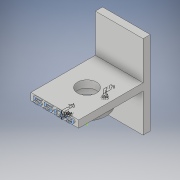
# Autodesk Inventor part: RSL mount
Saved by Autodesk Inventor 2019 (Build 230136000, 136)
## iProperties
Created: 2019-02-11
Part Number: RSL mount
Material: Generic
Document SubType Name: Modeling
Designer: josh
Density: 1 g/cm^3
Appearance: Default
Author: josh
Autodesk Inventor part; units mm, degrees
ref_plane "XZ Plane" through (0, 0, 0) normal (0, 1, 0) x (-1, 0, 0)
ref_plane "XY Plane" through (0, 0, 0) normal (0, 0, 1) x (1, 0, 0)
sketch "Sketch1" plane through (0, 0, 0) normal (0, 0, 1) x (1, 0, 0)
  line L0 (0, 0) -> (50.8, 0)
  line L1 (50.8, 0) -> (50.8, 88.9)
  line L2 (50.8, 88.9) -> (0, 88.9)
  line L3 (0, 88.9) -> (0, 0)
  line L4 (0, 88.9) -> (0, 48.26)
  line L5 (0, 0) -> (0, 40.64)
  line L6 (0, 40.64) -> (50.8, 40.64)
  line L7 (50.8, 48.26) -> (0, 48.26)
  dimension "d0" = 50.8
  dimension "d1" = 88.9
  dimension "d2" = 40.64
  dimension "d3" = 40.64
  constraints: 16 end point, 4 point on line, 3 perpendicular, 2 parallel, 1 horizontal
  measures "d0" distance of L2.end L1.end
  measures "d1" distance of L1.end L0.end
  measures "d2" distance of L2.end L4.end
  measures "d3" distance of L0.start L5.end
extrude "Extrusion1" add sketch "Sketch1" along normal blind 7.62
extrude "Extrusion2" add sketch "Sketch1" along normal blind 76.2 contours L3 L7 L1 L6
sketch "Sketch3" plane through (0, 48.26, 7.62) normal (0, 1, 0) x (1, 0, 0)
  line L0 (0, 0) -> (0, -68.58) projected
  line L1 (0, -34.29) -> (50.8, -34.29)
  line L2 (50.8, 0) -> (50.8, -68.58) projected
  circle A0 centre (25.4, -34.29) radius 10.16
  point P0 (0, 7.62)
  dimension "d8" = 20.32
  constraints: 3 midpoint, 2 end point, 1 centre point
  measures "d8" diameter of A0
extrude "Extrusion3" cut sketch "Sketch3" against normal blind 50.8
sketch "Sketch4" plane through (0, 0, 76.2) normal (0, 0, 1) x (1, 0, 0)
  line L0 (2.1147, 47.7276) -> (47.8791, 47.7276) construction
  line L1 (47.8791, 47.7276) -> (47.8791, 41.3797) construction
  line L2 (47.8791, 41.3797) -> (2.1147, 41.3797) construction
  line L3 (2.1147, 41.3797) -> (2.1147, 47.7276) construction
  spline S0 degree 2 poles (12.464, 43.4446) (12.464, 43.005) (11.7576, 42.2541) (11.1253, 41.9774) knots 0 0 0 1 2 2 2
  spline S1 degree 2 poles (11.1253, 41.9774) (10.4781, 41.7008) (8.5664, 41.3797) (7.3758, 41.3797) knots 0 0 0 1 2 2 2
  spline S2 degree 2 poles (7.3758, 41.3797) (6.2791, 41.3797) (4.1598, 41.5724) (3.3843, 41.7255) knots 0 0 0 1 2 2 2
  line L4 (3.3843, 41.7255) -> (3.3843, 42.59)
  line L5 (3.3843, 42.59) -> (3.5275, 42.59)
  spline S3 degree 2 poles (3.5275, 42.59) (3.7646, 42.5208) (4.644, 42.343) (5.1775, 42.264) knots 0 0 0 1 2 2 2
  spline S4 degree 2 poles (5.1775, 42.264) (5.7802, 42.18) (6.783, 42.0861) (7.4054, 42.0861) knots 0 0 0 1 2 2 2
  spline S5 degree 2 poles (7.4054, 42.0861) (8.018, 42.0861) (9.1888, 42.264) (9.6087, 42.4566) knots 0 0 0 1 2 2 2
  spline S6 degree 2 poles (9.6087, 42.4566) (9.9841, 42.6394) (10.3843, 43.1235) (10.3843, 43.4496) knots 0 0 0 1 2 2 2
  spline S7 degree 2 poles (10.3843, 43.4496) (10.3843, 43.7756) (9.9446, 44.1906) (9.5247, 44.3289) knots 0 0 0 1 2 2 2
  spline S8 degree 2 poles (9.5247, 44.3289) (9.0851, 44.482) (7.8056, 44.6105) (7.0152, 44.6105) knots 0 0 0 1 2 2 2
  spline S9 degree 2 poles (7.0152, 44.6105) (6.1853, 44.6105) (4.5106, 44.5067) (4.0067, 44.4623) knots 0 0 0 1 2 2 2
  line L6 (4.0067, 44.4623) -> (4.0067, 47.6041)
  line L7 (4.0067, 47.6041) -> (12.3702, 47.6041)
  line L8 (12.3702, 47.6041) -> (12.3702, 46.8878)
  line L9 (12.3702, 46.8878) -> (5.9827, 46.8878)
  line L10 (5.9827, 46.8878) -> (5.9827, 45.2626)
  spline S10 degree 2 poles (5.9827, 45.2626) (6.3532, 45.2823) (7.0695, 45.2971) (7.3659, 45.2971) knots 0 0 0 1 2 2 2
  spline S11 degree 2 poles (7.3659, 45.2971) (8.5318, 45.2971) (10.1521, 45.144) (10.898, 44.9168) knots 0 0 0 1 2 2 2
  spline S12 degree 2 poles (10.898, 44.9168) (11.6539, 44.6895) (12.464, 43.9979) (12.464, 43.4446) knots 0 0 0 1 2 2 2
  spline S13 degree 2 poles (23.9052, 43.4446) (23.9052, 43.005) (23.1987, 42.2541) (22.5664, 41.9774) knots 0 0 0 1 2 2 2
  spline S14 degree 2 poles (22.5664, 41.9774) (21.9193, 41.7008) (20.0075, 41.3797) (18.8169, 41.3797) knots 0 0 0 1 2 2 2
  spline S15 degree 2 poles (18.8169, 41.3797) (17.7202, 41.3797) (15.601, 41.5724) (14.8254, 41.7255) knots 0 0 0 1 2 2 2
  line L11 (14.8254, 41.7255) -> (14.8254, 42.59)
  line L12 (14.8254, 42.59) -> (14.9686, 42.59)
  spline S16 degree 2 poles (14.9686, 42.59) (15.2058, 42.5208) (16.0851, 42.343) (16.6186, 42.264) knots 0 0 0 1 2 2 2
  spline S17 degree 2 poles (16.6186, 42.264) (17.2213, 42.18) (18.2241, 42.0861) (18.8466, 42.0861) knots 0 0 0 1 2 2 2
  spline S18 degree 2 poles (18.8466, 42.0861) (19.4591, 42.0861) (20.6299, 42.264) (21.0498, 42.4566) knots 0 0 0 1 2 2 2
  spline S19 degree 2 poles (21.0498, 42.4566) (21.4253, 42.6394) (21.8254, 43.1235) (21.8254, 43.4496) knots 0 0 0 1 2 2 2
  spline S20 degree 2 poles (21.8254, 43.4496) (21.8254, 43.7756) (21.3857, 44.1906) (20.9658, 44.3289) knots 0 0 0 1 2 2 2
  spline S21 degree 2 poles (20.9658, 44.3289) (20.5262, 44.482) (19.2467, 44.6105) (18.4563, 44.6105) knots 0 0 0 1 2 2 2
  spline S22 degree 2 poles (18.4563, 44.6105) (17.6264, 44.6105) (15.9517, 44.5067) (15.4478, 44.4623) knots 0 0 0 1 2 2 2
  line L13 (15.4478, 44.4623) -> (15.4478, 47.6041)
  line L14 (15.4478, 47.6041) -> (23.8113, 47.6041)
  line L15 (23.8113, 47.6041) -> (23.8113, 46.8878)
  line L16 (23.8113, 46.8878) -> (17.4238, 46.8878)
  line L17 (17.4238, 46.8878) -> (17.4238, 45.2626)
  spline S23 degree 2 poles (17.4238, 45.2626) (17.7943, 45.2823) (18.5106, 45.2971) (18.807, 45.2971) knots 0 0 0 1 2 2 2
  spline S24 degree 2 poles (18.807, 45.2971) (19.9729, 45.2971) (21.5932, 45.144) (22.3392, 44.9168) knots 0 0 0 1 2 2 2
  spline S25 degree 2 poles (22.3392, 44.9168) (23.095, 44.6895) (23.9052, 43.9979) (23.9052, 43.4446) knots 0 0 0 1 2 2 2
  spline S26 degree 2 poles (35.5883, 44.5561) (35.5883, 42.9161) (33.2023, 41.3797) (30.7175, 41.3797) knots 0 0 0 1 2 2 2
  spline S27 degree 2 poles (30.7175, 41.3797) (28.198, 41.3797) (25.8466, 42.9457) (25.8466, 44.5512) knots 0 0 0 1 2 2 2
  spline S28 degree 2 poles (25.8466, 44.5512) (25.8466, 46.2012) (28.2326, 47.7276) (30.7175, 47.7276) knots 0 0 0 1 2 2 2
  spline S29 degree 2 poles (30.7175, 47.7276) (33.2369, 47.7276) (35.5883, 46.1468) (35.5883, 44.5561) knots 0 0 0 1 2 2 2
  spline S30 degree 2 poles (32.9652, 42.6987) (33.2616, 43) (33.5086, 43.9288) (33.5086, 44.5561) knots 0 0 0 1 2 2 2
  spline S31 degree 2 poles (33.5086, 44.5561) (33.5086, 45.1835) (33.2616, 46.1073) (32.9553, 46.4185) knots 0 0 0 1 2 2 2
  spline S32 degree 2 poles (32.9553, 46.4185) (32.649, 46.7298) (31.577, 47.0509) (30.7175, 47.0509) knots 0 0 0 1 2 2 2
  spline S33 degree 2 poles (30.7175, 47.0509) (29.8678, 47.0509) (28.776, 46.7298) (28.4599, 46.4087) knots 0 0 0 1 2 2 2
  spline S34 degree 2 poles (28.4599, 46.4087) (28.1536, 46.0974) (27.9263, 45.1489) (27.9263, 44.5512) knots 0 0 0 1 2 2 2
  spline S35 degree 2 poles (27.9263, 44.5512) (27.9263, 43.909) (28.119, 43.0494) (28.45, 42.7135) knots 0 0 0 1 2 2 2
  spline S36 degree 2 poles (28.45, 42.7135) (28.7464, 42.3973) (29.8381, 42.0565) (30.7175, 42.0565) knots 0 0 0 1 2 2 2
  spline S37 degree 2 poles (30.7175, 42.0565) (31.5671, 42.0565) (32.6589, 42.3776) (32.9652, 42.6987) knots 0 0 0 1 2 2 2
  spline S38 degree 2 poles (37.1247, 45.6232) (37.1247, 46.0925) (37.8904, 46.873) (38.5573, 47.1546) knots 0 0 0 1 2 2 2
  spline S39 degree 2 poles (38.5573, 47.1546) (39.1896, 47.4263) (41.0224, 47.7276) (41.9659, 47.7276) knots 0 0 0 1 2 2 2
  spline S40 degree 2 poles (41.9659, 47.7276) (43.0181, 47.7276) (44.7274, 47.4461) (45.3498, 47.1793) knots 0 0 0 1 2 2 2
  spline S41 degree 2 poles (45.3498, 47.1793) (46.1402, 46.8434) (47.0097, 45.7566) (47.0097, 44.9217) knots 0 0 0 1 2 2 2
  spline S42 degree 2 poles (47.0097, 44.9217) (47.0097, 44.1659) (46.16, 42.8123) (45.3301, 42.3628) knots 0 0 0 1 2 2 2
  spline S43 degree 2 poles (45.3301, 42.3628) (44.4507, 41.8885) (41.9857, 41.3896) (40.1727, 41.3896) knots 0 0 0 1 2 2 2
  spline S44 degree 2 poles (40.1727, 41.3896) (39.7627, 41.3896) (38.8438, 41.4242) (38.4437, 41.4736) knots 0 0 0 1 2 2 2
  line L18 (38.4437, 41.4736) -> (38.4437, 42.259)
  line L19 (38.4437, 42.259) -> (38.5474, 42.259)
  spline S45 degree 2 poles (38.5474, 42.259) (38.8043, 42.1997) (39.8862, 42.096) (40.4493, 42.096) knots 0 0 0 1 2 2 2
  spline S46 degree 2 poles (40.4493, 42.096) (42.455, 42.096) (44.7521, 43.1532) (44.9052, 44.1313) knots 0 0 0 1 2 2 2
  spline S47 degree 2 poles (44.9052, 44.1313) (44.0852, 43.909) (42.5982, 43.7065) (41.7288, 43.7065) knots 0 0 0 1 2 2 2
  spline S48 degree 2 poles (41.7288, 43.7065) (40.8791, 43.7065) (39.491, 43.8547) (38.7845, 44.0671) knots 0 0 0 1 2 2 2
  spline S49 degree 2 poles (38.7845, 44.0671) (37.9645, 44.319) (37.1247, 45.0847) (37.1247, 45.6232) knots 0 0 0 1 2 2 2
  spline S50 degree 2 poles (44.9546, 45.1045) (44.9546, 45.722) (44.3816, 46.5025) (43.8826, 46.7149) knots 0 0 0 1 2 2 2
  spline S51 degree 2 poles (43.8826, 46.7149) (43.4282, 46.9125) (42.5093, 47.0607) (41.956, 47.0607) knots 0 0 0 1 2 2 2
  spline S52 degree 2 poles (41.956, 47.0607) (40.6963, 47.0607) (39.2044, 46.3395) (39.2044, 45.6578) knots 0 0 0 1 2 2 2
  spline S53 degree 2 poles (39.2044, 45.6578) (39.2044, 45.2724) (39.6935, 44.7735) (40.2468, 44.5957) knots 0 0 0 1 2 2 2
  spline S54 degree 2 poles (40.2468, 44.5957) (40.637, 44.4672) (41.6201, 44.3832) (42.1833, 44.3832) knots 0 0 0 1 2 2 2
  spline S55 degree 2 poles (42.1833, 44.3832) (42.8354, 44.3832) (44.3519, 44.566) (44.9151, 44.7192) knots 0 0 0 1 2 2 2
  spline S56 degree 2 poles (44.9151, 44.7192) (44.925, 44.7784) (44.9546, 44.981) (44.9546, 45.1045) knots 0 0 0 1 2 2 2
  point P0 (0, 0)
  constraints: 2 other
emboss "Emboss1" sketch "Sketch4" operation add depth 1.27 direction (0, 0, -1)
ref_plane "Work Plane1" through (25.4, 0, 0) normal (1, 0, 0) x (0, 1, 0)
sketch "Sketch5" plane through (25.4, 0, 0) normal (1, 0, 0) x (0, 1, 0)
  line L0 (40.64, 56.014) -> (32.131, 56.014)
  line L1 (40.64, 27.806) -> (32.131, 27.806)
  line L2 (40.64, 56.014) -> (40.64, 62.364)
  line L3 (32.131, 62.364) -> (32.131, 56.014)
  line L4 (32.131, 27.806) -> (32.131, 21.456)
  line L5 (32.131, 62.364) -> (36.3855, 62.364)
  line L6 (36.3855, 62.364) -> (36.3855, 61.094)
  line L7 (36.3855, 61.094) -> (33.8455, 61.094)
  line L8 (33.8455, 61.094) -> (33.8455, 59.189)
  line L9 (33.8455, 59.189) -> (38.1635, 59.189)
  line L10 (38.1635, 59.189) -> (38.1635, 62.364)
  line L11 (38.1635, 21.456) -> (38.1635, 24.631)
  line L12 (38.1635, 24.631) -> (33.8455, 24.631)
  line L13 (33.8455, 24.631) -> (33.8455, 22.726)
  line L14 (33.8455, 22.726) -> (36.3855, 22.726)
  line L15 (36.3855, 22.726) -> (36.3855, 21.456)
  line L16 (40.64, 41.91) -> (13.3619, 41.91)
  line L17 (40.64, 21.456) -> (38.1635, 21.456)
  line L18 (36.3855, 21.456) -> (32.131, 21.456)
  line L19 (40.64, 62.364) -> (38.1635, 62.364)
  line L20 (36.3855, 62.364) -> (32.131, 62.364)
  line L21 (40.64, 21.456) -> (40.64, 27.806)
  point P0 (0, 0)
  dimension "d15" = 8.509
  dimension "d18" = 6.35
  dimension "d19" = 1.27
  dimension "d20" = 2.54
  dimension "d21" = 4.318
  dimension "d22" = 3.175
  dimension "d23" = 4.318
  dimension "d25" = 1.27
  constraints: 44 end point, 8 perpendicular, 3 vertical, 2 horizontal, 1 collinear, 1 parallel
  measures "d15" distance of L0.start L0.end
  measures "d18" distance of L0.start L2.end
  measures "d19" distance of L5.end L6.end
  measures "d20" distance of L6.end L7.end
  measures "d21" distance of L8.end L9.end
  measures "d22" distance of L11.start L11.end
  measures "d23" distance of L11.end L12.end
  measures "d25" distance of L14.end L15.end
revolve "Revolution1" add sketch "Sketch5" angle 15 about axis through (25.4, 40.64, 41.91) along (0, -1, 0)
ref_plane "Work Plane2" through (20.1061, 38.1635, 61.667) normal (-0.9659258, 0, -0.258819) x (0, -1, 0)
sketch "Sketch6" plane through (20.1061, 38.1635, 61.667) normal (-0.9659258, 0, -0.258819) x (0, -1, 0)
  line L0 (-2.4765, -6.35) -> (-2.4765, 0) projected
  line L1 (-2.4765, -6.35) -> (6.0325, -6.35) projected
  line L2 (6.0325, -6.35) -> (6.0325, 0) projected
  line L3 (6.0325, 0) -> (1.778, 0) projected
  line L4 (1.778, 0) -> (1.778, -1.27) projected
  line L5 (1.778, -1.27) -> (4.318, -1.27) projected
  line L6 (4.318, -1.27) -> (4.318, -3.175) projected
  line L7 (4.318, -3.175) -> (0, -3.175) projected
  line L8 (0, -3.175) -> (0, 0) projected
  line L9 (0, 0) -> (-2.4765, 0) projected
  line L10 (1.778, 0) -> (1.778, -1.27) projected
  line L11 (1.778, -1.27) -> (1.778, -3.175)
  line L12 (1.778, 0) -> (1.778, -1.27)
  line L13 (-2.4765, -6.35) -> (6.0325, -6.35)
  line L14 (6.0325, -6.35) -> (6.0325, 0)
  line L15 (-2.4765, 0) -> (-2.4765, -6.35)
  line L16 (6.0325, 0) -> (1.778, 0)
  line L17 (0, 0) -> (-2.4765, 0)
  line L18 (0, -3.175) -> (0, 0) projected
  line L19 (1.778, -3.175) -> (0, -3.175)
  line L20 (0, -3.175) -> (0, 0)
  line L21 (-2.4765, -34.558) -> (6.0325, -34.558) projected
  line L22 (6.0325, -34.558) -> (6.0325, -40.908) projected
  line L23 (6.0325, -40.908) -> (1.778, -40.908) projected
  line L24 (1.778, -40.908) -> (1.778, -39.638) projected
  line L25 (1.778, -39.638) -> (4.318, -39.638) projected
  line L26 (4.318, -39.638) -> (4.318, -37.733) projected
  line L27 (4.318, -37.733) -> (0, -37.733) projected
  line L28 (0, -37.733) -> (0, -40.908) projected
  line L29 (0, -40.908) -> (-2.4765, -40.908) projected
  line L30 (-2.4765, -34.558) -> (-2.4765, -40.908) projected
  line L31 (1.778, -40.908) -> (1.778, -37.733)
  line L32 (4.318, -37.733) -> (0, -37.733) projected
  line L33 (1.778, -37.733) -> (0, -37.733)
  line L34 (0, -37.733) -> (0, -40.908)
  line L35 (-2.4765, -34.558) -> (6.0325, -34.558)
  line L36 (6.0325, -34.558) -> (6.0325, -40.908)
  line L37 (-2.4765, -40.908) -> (-2.4765, -34.558)
  line L38 (6.0325, -40.908) -> (1.778, -40.908)
  line L39 (0, -40.908) -> (-2.4765, -40.908)
  line L40 (-2.4765, 0) -> (-2.4765, -40.908)
  line L41 (-2.4765, -47.0016) -> (-2.4765, 19.2416) projected
  line L42 (-2.4765, -20.454) -> (9.1387, -20.454)
  point P0 (38.1635, -54.3619)
  constraints: 39 end point, 6 parallel, 6 perpendicular, 4 horizontal, 2 collinear, 2 point on line, 1 midpoint, 1 vertical
revolve "Revolution2" add sketch "Sketch6" angle 20 about axis through (25.4, 40.64, 41.91) along (0, -1, 0)
ref_plane "Work Plane3" through (25.4, 36.3855, 62.364) normal (-1, 0, 0) x (0, -1, 0)
sketch "Sketch7" plane through (25.4, 36.3855, 62.364) normal (-1, 0, 0) x (0, -1, 0)
  line L0 (-4.2545, 0) -> (-4.2545, -6.35) projected
  line L1 (-4.2545, 0) -> (-1.778, 0) projected
  line L2 (0, 0) -> (4.2545, 0) projected
  line L3 (4.2545, 0) -> (4.2545, -6.35) projected
  line L4 (4.2545, -6.35) -> (-4.2545, -6.35) projected
  line L5 (-4.2545, -34.558) -> (4.2545, -34.558) projected
  line L6 (-4.2545, -40.908) -> (-4.2545, -34.558) projected
  line L7 (-1.778, -40.908) -> (-4.2545, -40.908) projected
  line L8 (4.2545, -40.908) -> (0, -40.908) projected
  line L9 (4.2545, -34.558) -> (4.2545, -40.908) projected
  line L10 (-4.2545, 0) -> (4.2545, 0)
  line L11 (4.2545, 0) -> (4.2545, -6.35)
  line L12 (4.2545, -6.35) -> (-4.2545, -6.35)
  line L13 (-4.2545, -6.35) -> (-4.2545, 0)
  line L14 (-4.2545, -40.908) -> (4.2545, -40.908)
  line L15 (4.2545, -40.908) -> (4.2545, -34.558)
  line L16 (4.2545, -34.558) -> (-4.2545, -34.558)
  line L17 (-4.2545, -34.558) -> (-4.2545, -40.908)
  line L18 (-4.2545, -40.908) -> (-4.2545, 0)
  line L19 (-4.2545, -20.454) -> (4.2545, -20.454)
  point P0 (36.3855, -62.364)
  point P1 (-1.778, -3.175)
  constraints: 20 end point, 4 parallel, 3 horizontal, 2 perpendicular, 1 midpoint, 1 vertical
revolve "Revolution3" add sketch "Sketch7" angle 130 about axis through (25.4, 40.64, 41.91) along (0, 1, 0)
ref_plane "Work Plane4" through (13.6681, 36.3855, 58.6649) normal (-0.819152, 0, -0.5735764) x (0, -1, 0)
sketch "Sketch8" plane through (13.6681, 36.3855, 58.6649) normal (-0.819152, 0, -0.5735764) x (0, -1, 0)
  line L0 (0, -3.175) -> (-1.778, -3.175) projected
  line L1 (-1.778, -3.175) -> (-1.778, 0) projected
  line L2 (-1.778, 0) -> (-4.2545, 0) projected
  line L3 (-4.2545, -6.35) -> (-4.2545, 0) projected
  line L4 (-4.2545, -6.35) -> (4.2545, -6.35) projected
  line L5 (4.2545, -6.35) -> (4.2545, 0) projected
  line L6 (4.2545, 0) -> (0, 0) projected
  line L7 (0, 0) -> (0, -3.175) projected
  line L8 (0, -40.908) -> (0, -37.733) projected
  line L9 (0, -37.733) -> (-1.778, -37.733) projected
  line L10 (-1.778, -37.733) -> (-1.778, -40.908) projected
  line L11 (-1.778, -40.908) -> (-4.2545, -40.908) projected
  line L12 (-4.2545, -34.558) -> (-4.2545, -40.908) projected
  line L13 (-4.2545, -34.558) -> (4.2545, -34.558) projected
  line L14 (4.2545, -34.558) -> (4.2545, -40.908) projected
  line L15 (4.2545, -40.908) -> (0, -40.908) projected
  line L16 (-1.778, -37.733) -> (-1.778, -34.6081) projected
  line L17 (-1.778, -37.733) -> (4.2545, -37.733)
  line L18 (4.2545, -34.558) -> (-4.2545, -34.558)
  line L19 (4.2545, -40.908) -> (0, -40.908) projected
  line L20 (-4.2545, -34.558) -> (-4.2545, -40.908) projected
  line L21 (-4.2545, -40.908) -> (-1.778, -40.908)
  line L22 (-1.778, -37.733) -> (-1.778, -40.908)
  line L23 (-4.2545, -6.35) -> (4.2545, -6.35) projected
  line L24 (4.2545, -6.35) -> (-4.2545, -6.35)
  line L25 (-4.2545, -6.35) -> (-4.2545, 0)
  line L26 (-1.778, 0) -> (-1.778, -3.175)
  line L27 (0, -3.175) -> (-1.778, -3.175) projected
  line L28 (-1.778, -3.175) -> (4.2545, -3.175)
  line L29 (4.2545, -6.35) -> (4.2545, 0) projected
  line L30 (4.2545, -3.175) -> (4.2545, -6.35)
  line L31 (-1.778, -40.908) -> (-4.2545, -40.908) projected
  line L32 (-4.2545, -40.908) -> (-4.2545, 0)
  line L33 (-4.2545, -20.454) -> (21.1387, -20.454)
  point P0 (36.3855, -40.2158)
  constraints: 22 end point, 3 collinear, 3 midpoint, 3 perpendicular, 1 horizontal, 1 parallel
revolve "Revolution4" add sketch "Sketch8" angle 15 about axis through (25.4, 40.64, 41.91) along (0, -1, 0) contours L28 L5 L4 L3 L2 L1 L0 | L9 L10 L11 L12 L13 L14 L17
body "Solid1"
